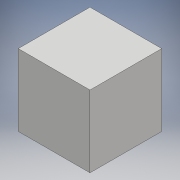
# Autodesk Inventor part: CalibrationCube
Saved by Autodesk Inventor 2017 (Build 210142000, 142)
## iProperties
Created: 2018-12-06
Part Number: CalibrationCube
Material: Generic
Document SubType Name: Modeling
Designer: Eric the Great
Density: 1 g/cm^3
Appearance: Default
Author: Eric the Great
Autodesk Inventor part; units mm, degrees
ref_plane "YZ Plane" through (0, 0, 0) normal (1, 0, 0) x (0, 1, 0)
ref_plane "XZ Plane" through (0, 0, 0) normal (0, 1, 0) x (-1, 0, 0)
ref_plane "XY Plane" through (0, 0, 0) normal (0, 0, 1) x (1, 0, 0)
sketch "Sketch1" plane through (0, 0, 0) normal (0, 1, 0) x (-1, 0, 0)
  line L0 (-28.325, 28.325) -> (28.325, 28.325)
  line L1 (28.325, 28.325) -> (28.325, -28.325)
  line L2 (28.325, -28.325) -> (-28.325, -28.325)
  line L3 (-28.325, -28.325) -> (-28.325, 28.325)
  line L4 (-28.325, 28.325) -> (28.325, -28.325) construction
  line L5 (28.325, 28.325) -> (-28.325, -28.325) construction
  point P0 (0, 0)
  dimension "d1" = 56.65
  constraints: 12 end point, 2 midpoint, 2 parallel, 2 perpendicular, 1 horizontal
  measures "d1" distance of L0.end L1.end
extrude "Extrusion1" add sketch "Sketch1" along normal blind 56.65
sketch "Sketch2" plane through (0, 56.65, 0) normal (0, 1, 0) x (1, 0, 0)
  line L0 (-12.2741, -17.9438) -> (-12.2741, 26.8853) construction
  line L1 (-12.2741, 26.8853) -> (-6.3057, 26.8853) construction
  line L2 (-6.3057, 26.8853) -> (-6.3057, -17.9438) construction
  line L3 (-6.3057, -17.9438) -> (-12.2741, -17.9438) construction
  line L4 (-0.0592, -21.5544) -> (-0.0592, 23.2747) construction
  line L5 (-0.0592, 23.2747) -> (5.9092, 23.2747) construction
  line L6 (5.9092, 23.2747) -> (5.9092, -21.5544) construction
  line L7 (5.9092, -21.5544) -> (-0.0592, -21.5544) construction
  line L8 (-6.8824, -13.4747) -> (-6.8824, -14.3929)
  line L9 (-6.8824, -14.3929) -> (-9.0147, -15.8246)
  line L10 (-9.0147, -15.8246) -> (-9.0147, -16.5513)
  line L11 (-9.0147, -16.5513) -> (-6.8824, -16.5513)
  line L12 (-6.8824, -16.5513) -> (-6.8824, -17.2954)
  line L13 (-6.8824, -17.2954) -> (-11.8824, -17.2954)
  line L14 (-11.8824, -17.2954) -> (-11.8824, -15.5417)
  spline S0 degree 2 poles (-11.8824, -15.5417) (-11.8824, -14.6018) (-11.5038, -13.7837) (-10.9033, -13.7837) knots 0 0 0 1 2 2 2
  line L15 (-10.9033, -13.7837) -> (-10.0417, -13.7837)
  spline S1 degree 2 poles (-10.0417, -13.7837) (-9.5804, -13.7837) (-9.1105, -14.5409) (-9.1105, -15.0805) knots 0 0 0 1 2 2 2
  line L16 (-9.1105, -15.0805) -> (-6.8824, -13.4747)
  line L17 (-10.1331, -14.5322) -> (-10.825, -14.5322)
  spline S2 degree 2 poles (-10.825, -14.5322) (-11.3864, -14.5322) (-11.3864, -15.5026) knots 0 0 0 1 1 1
  line L18 (-11.3864, -15.5026) -> (-11.3864, -16.5513)
  line L19 (-11.3864, -16.5513) -> (-9.5108, -16.5513)
  line L20 (-9.5108, -16.5513) -> (-9.5108, -15.5722)
  spline S3 degree 2 poles (-9.5108, -15.5722) (-9.5108, -15.0413) (-9.7719, -14.5322) (-10.1331, -14.5322) knots 0 0 0 1 2 2 2
  line L21 (-9.3541, -9.332) -> (-8.0617, -9.332)
  spline S4 degree 2 poles (-8.0617, -9.332) (-7.7136, -9.332) (-7.2349, -9.5017) (-6.9738, -9.7628) (-6.8346, -10.2502) (-6.8041, -10.6897) (-6.8041, -11.0509) knots 0 0 0 1 2 3 4 5 5 5
  spline S5 degree 2 poles (-6.8041, -11.0509) (-6.8041, -11.5122) (-6.865, -12.03) (-7.1044, -12.5435) (-7.6309, -12.7698) (-8.0617, -12.7698) knots 0 0 0 1 2 3 4 4 4
  line L22 (-8.0617, -12.7698) -> (-9.3541, -12.7698)
  spline S6 degree 2 poles (-9.3541, -12.7698) (-9.724, -12.7698) (-10.2332, -12.5914) (-10.5117, -12.339) (-10.6553, -11.8429) (-10.6857, -11.4208) (-10.6857, -10.681) (-10.6553, -10.2589) (-10.5117, -9.7628) (-10.2332, -9.5104) (-9.724, -9.332) (-9.3541, -9.332) knots 0 0 0 1 2 3 4 5 6 7 8 9 10 10 10
  line L23 (-7.9616, -10.0413) -> (-9.4716, -10.0413)
  spline S7 degree 2 poles (-9.4716, -10.0413) (-9.9851, -10.0413) (-10.2332, -10.4591) (-10.2332, -11.6427) (-9.9851, -12.0605) (-9.4716, -12.0605) knots 0 0 0 1 2 3 4 4 4
  line L24 (-9.4716, -12.0605) -> (-7.9616, -12.0605)
  spline S8 degree 2 poles (-7.9616, -12.0605) (-7.7136, -12.0605) (-7.422, -11.9517) (-7.2915, -11.6601) (-7.261, -11.3511) (-7.261, -10.7506) (-7.2915, -10.4417) (-7.422, -10.1501) (-7.7136, -10.0413) (-7.9616, -10.0413) knots 0 0 0 1 2 3 4 5 6 7 8 8 8
  line L25 (-9.6327, -4.8585) -> (-8.1009, -4.8585)
  spline S9 degree 2 poles (-8.1009, -4.8585) (-7.7615, -4.8585) (-7.2697, -5.0587) (-6.9999, -5.359) (-6.8433, -5.8551) (-6.8041, -6.2859) (-6.8041, -6.5948) knots 0 0 0 1 2 3 4 5 5 5
  spline S10 degree 2 poles (-6.8041, -6.5948) (-6.8041, -6.9952) (-6.8824, -7.5) (-7.1305, -8.0091) (-7.6744, -8.2571) (-8.1009, -8.2571) knots 0 0 0 1 2 3 4 4 4
  line L26 (-8.1009, -8.2571) -> (-12.2741, -8.2571)
  line L27 (-12.2741, -8.2571) -> (-12.2741, -7.5652)
  line L28 (-12.2741, -7.5652) -> (-11.1557, -7.5652)
  spline S11 degree 2 poles (-11.1557, -7.5652) (-11.0121, -7.5652) (-10.4159, -7.5696) (-10.2723, -7.5696) knots 0 0 0 1 2 2 2
  spline S12 degree 2 poles (-10.2723, -7.5696) (-10.4508, -7.5391) (-10.6857, -6.9647) (-10.6857, -6.399) knots 0 0 0 1 2 2 2
  spline S13 degree 2 poles (-10.6857, -6.399) (-10.6857, -4.8585) (-9.6327, -4.8585) knots 0 0 0 1 1 1
  line L29 (-8.0008, -5.5679) -> (-9.4629, -5.5679)
  spline S14 degree 2 poles (-9.4629, -5.5679) (-9.9416, -5.5679) (-10.194, -6.0161) (-10.194, -6.5861) knots 0 0 0 1 2 2 2
  spline S15 degree 2 poles (-10.194, -6.5861) (-10.194, -7.1344) (-9.9025, -7.5652) (-9.4629, -7.5652) knots 0 0 0 1 2 2 2
  line L30 (-9.4629, -7.5652) -> (-8.0008, -7.5652)
  spline S16 degree 2 poles (-8.0008, -7.5652) (-7.5308, -7.5652) (-7.261, -7.1388) (-7.261, -6.5774) knots 0 0 0 1 2 2 2
  spline S17 degree 2 poles (-7.261, -6.5774) (-7.261, -6.0074) (-7.5308, -5.5679) (-8.0008, -5.5679) knots 0 0 0 1 2 2 2
  line L31 (-9.3541, -0.4982) -> (-8.0617, -0.4982)
  spline S18 degree 2 poles (-8.0617, -0.4982) (-7.7136, -0.4982) (-7.2349, -0.6679) (-6.9738, -0.929) (-6.8346, -1.4164) (-6.8041, -1.8559) (-6.8041, -2.2171) knots 0 0 0 1 2 3 4 5 5 5
  spline S19 degree 2 poles (-6.8041, -2.2171) (-6.8041, -2.6784) (-6.865, -3.1962) (-7.1044, -3.7097) (-7.6309, -3.936) (-8.0617, -3.936) knots 0 0 0 1 2 3 4 4 4
  line L32 (-8.0617, -3.936) -> (-9.3541, -3.936)
  spline S20 degree 2 poles (-9.3541, -3.936) (-9.724, -3.936) (-10.2332, -3.7576) (-10.5117, -3.5052) (-10.6553, -3.0091) (-10.6857, -2.587) (-10.6857, -1.8472) (-10.6553, -1.4251) (-10.5117, -0.929) (-10.2332, -0.6766) (-9.724, -0.4982) (-9.3541, -0.4982) knots 0 0 0 1 2 3 4 5 6 7 8 9 10 10 10
  line L33 (-7.9616, -1.2075) -> (-9.4716, -1.2075)
  spline S21 degree 2 poles (-9.4716, -1.2075) (-9.9851, -1.2075) (-10.2332, -1.6253) (-10.2332, -2.8089) (-9.9851, -3.2267) (-9.4716, -3.2267) knots 0 0 0 1 2 3 4 4 4
  line L34 (-9.4716, -3.2267) -> (-7.9616, -3.2267)
  spline S22 degree 2 poles (-7.9616, -3.2267) (-7.7136, -3.2267) (-7.422, -3.1179) (-7.2915, -2.8263) (-7.261, -2.5174) (-7.261, -1.9169) (-7.2915, -1.6079) (-7.422, -1.3163) (-7.7136, -1.2075) (-7.9616, -1.2075) knots 0 0 0 1 2 3 4 5 6 7 8 8 8
  spline S23 degree 2 poles (-6.9129, 3.2746) (-6.8041, 2.7655) (-6.8041, 2.0779) knots 0 0 0 1 1 1
  spline S24 degree 2 poles (-6.8041, 2.0779) (-6.8041, 1.7385) (-6.8302, 1.3643) (-6.9608, 0.8769) (-7.2045, 0.6245) (-7.6744, 0.4374) (-8.0226, 0.4374) knots 0 0 0 1 2 3 4 5 5 5
  line L35 (-8.0226, 0.4374) -> (-9.3933, 0.4374)
  spline S25 degree 2 poles (-9.3933, 0.4374) (-9.7023, 0.4374) (-10.1461, 0.5549) (-10.4246, 0.7986) (-10.5944, 1.064) (-10.664, 1.5166) (-10.6857, 1.8647) (-10.6857, 2.1563) knots 0 0 0 1 2 3 4 5 6 6 6
  spline S26 degree 2 poles (-10.6857, 2.1563) (-10.6857, 2.6872) (-10.5726, 3.218) knots 0 0 0 1 1 1
  line L36 (-10.5726, 3.218) -> (-10.0635, 3.218)
  spline S27 degree 2 poles (-10.0635, 3.218) (-10.2158, 2.6175) (-10.2158, 2.0692) knots 0 0 0 1 1 1
  spline S28 degree 2 poles (-10.2158, 2.0692) (-10.2158, 1.4948) (-9.9416, 1.1467) (-9.4934, 1.1467) knots 0 0 0 1 2 2 2
  line L37 (-9.4934, 1.1467) -> (-7.9703, 1.1467)
  spline S29 degree 2 poles (-7.9703, 1.1467) (-7.5613, 1.1467) (-7.2915, 1.5383) (-7.2915, 2.1476) knots 0 0 0 1 2 2 2
  spline S30 degree 2 poles (-7.2915, 2.1476) (-7.2915, 2.6959) (-7.4351, 3.2746) knots 0 0 0 1 1 1
  line L38 (-7.4351, 3.2746) -> (-6.9129, 3.2746)
  line L39 (-6.8824, 7.3608) -> (-6.8824, 6.6689)
  line L40 (-6.8824, 6.6689) -> (-7.335, 6.6689)
  spline S31 degree 2 poles (-7.335, 6.6689) (-6.8041, 6.5601) (-6.8041, 5.4417) knots 0 0 0 1 1 1
  spline S32 degree 2 poles (-6.8041, 5.4417) (-6.8041, 4.7063) (-7.335, 4.1493) (-7.8746, 4.1493) knots 0 0 0 1 2 2 2
  line L41 (-7.8746, 4.1493) -> (-10.6118, 4.1493)
  line L42 (-10.6118, 4.1493) -> (-10.6118, 4.8412)
  line L43 (-10.6118, 4.8412) -> (-7.9138, 4.8412)
  spline S33 degree 2 poles (-7.9138, 4.8412) (-7.7745, 4.8412) (-7.5917, 4.8891) (-7.4003, 5.037) (-7.3002, 5.3808) (-7.3002, 5.6419) knots 0 0 0 1 2 3 4 4 4
  spline S34 degree 2 poles (-7.3002, 5.6419) (-7.3002, 6.2207) (-7.5134, 6.6689) (-7.8006, 6.6689) knots 0 0 0 1 2 2 2
  line L44 (-7.8006, 6.6689) -> (-10.6118, 6.6689)
  line L45 (-10.6118, 6.6689) -> (-10.6118, 7.3608)
  line L46 (-10.6118, 7.3608) -> (-6.8824, 7.3608)
  line L47 (-9.6327, 11.9604) -> (-8.1009, 11.9604)
  spline S35 degree 2 poles (-8.1009, 11.9604) (-7.7615, 11.9604) (-7.2697, 11.7603) (-6.9999, 11.46) (-6.8433, 10.9639) (-6.8041, 10.5331) (-6.8041, 10.2241) knots 0 0 0 1 2 3 4 5 5 5
  spline S36 degree 2 poles (-6.8041, 10.2241) (-6.8041, 9.8238) (-6.8824, 9.319) (-7.1305, 8.8099) (-7.6744, 8.5618) (-8.1009, 8.5618) knots 0 0 0 1 2 3 4 4 4
  line L48 (-8.1009, 8.5618) -> (-12.2741, 8.5618)
  line L49 (-12.2741, 8.5618) -> (-12.2741, 9.2537)
  line L50 (-12.2741, 9.2537) -> (-11.1557, 9.2537)
  spline S37 degree 2 poles (-11.1557, 9.2537) (-11.0121, 9.2537) (-10.4159, 9.2494) (-10.2723, 9.2494) knots 0 0 0 1 2 2 2
  spline S38 degree 2 poles (-10.2723, 9.2494) (-10.4508, 9.2798) (-10.6857, 9.8543) (-10.6857, 10.42) knots 0 0 0 1 2 2 2
  spline S39 degree 2 poles (-10.6857, 10.42) (-10.6857, 11.9604) (-9.6327, 11.9604) knots 0 0 0 1 1 1
  line L51 (-8.0008, 11.2511) -> (-9.4629, 11.2511)
  spline S40 degree 2 poles (-9.4629, 11.2511) (-9.9416, 11.2511) (-10.194, 10.8029) (-10.194, 10.2328) knots 0 0 0 1 2 2 2
  spline S41 degree 2 poles (-10.194, 10.2328) (-10.194, 9.6845) (-9.9025, 9.2537) (-9.4629, 9.2537) knots 0 0 0 1 2 2 2
  line L52 (-9.4629, 9.2537) -> (-8.0008, 9.2537)
  spline S42 degree 2 poles (-8.0008, 9.2537) (-7.5308, 9.2537) (-7.261, 9.6802) (-7.261, 10.2415) knots 0 0 0 1 2 2 2
  spline S43 degree 2 poles (-7.261, 10.2415) (-7.261, 10.8116) (-7.5308, 11.2511) (-8.0008, 11.2511) knots 0 0 0 1 2 2 2
  line L53 (-8.5926, 16.0901) -> (-8.5926, 13.5836)
  line L54 (-8.5926, 13.5836) -> (-8.0313, 13.5836)
  spline S44 degree 2 poles (-8.0313, 13.5836) (-7.6353, 13.5836) (-7.3045, 14.1406) (-7.3045, 14.6845) knots 0 0 0 1 2 2 2
  spline S45 degree 2 poles (-7.3045, 14.6845) (-7.3045, 15.2198) (-7.4917, 15.9422) knots 0 0 0 1 1 1
  line L55 (-7.4917, 15.9422) -> (-6.9608, 15.9422)
  spline S46 degree 2 poles (-6.9608, 15.9422) (-6.8041, 15.2502) (-6.8041, 14.5932) knots 0 0 0 1 1 1
  spline S47 degree 2 poles (-6.8041, 14.5932) (-6.8041, 12.883) (-7.9442, 12.883) knots 0 0 0 1 1 1
  line L56 (-7.9442, 12.883) -> (-9.4151, 12.883)
  spline S48 degree 2 poles (-9.4151, 12.883) (-10.1026, 12.883) (-10.6857, 13.6706) (-10.6857, 14.5322) knots 0 0 0 1 2 2 2
  spline S49 degree 2 poles (-10.6857, 14.5322) (-10.6857, 15.3416) (-10.1244, 16.0901) (-9.4151, 16.0901) knots 0 0 0 1 2 2 2
  line L57 (-9.4151, 16.0901) -> (-8.5926, 16.0901)
  line L58 (-9.0452, 15.3939) -> (-9.6327, 15.3939)
  spline S50 degree 2 poles (-9.6327, 15.3939) (-9.9721, 15.3939) (-10.2245, 14.9804) (-10.2245, 14.4931) knots 0 0 0 1 2 2 2
  spline S51 degree 2 poles (-10.2245, 14.4931) (-10.2245, 14.0318) (-9.9808, 13.5836) (-9.6327, 13.5836) knots 0 0 0 1 2 2 2
  line L59 (-9.6327, 13.5836) -> (-9.0452, 13.5836)
  line L60 (-9.0452, 13.5836) -> (-9.0452, 15.3939)
  line L61 (1.5257, 0.3275) -> (2.4447, 0.3275)
  spline S52 degree 2 poles (2.4447, 0.3275) (2.6484, 0.3275) (2.9434, 0.2074) (3.1053, 0.0273) (3.1993, -0.2704) (3.2228, -0.5289) (3.2228, -0.7142) knots 0 0 0 1 2 3 4 5 5 5
  spline S53 degree 2 poles (3.2228, -0.7142) (3.2228, -0.9545) (3.1758, -1.2573) (3.027, -1.5628) (2.7006, -1.7116) (2.4447, -1.7116) knots 0 0 0 1 2 3 4 4 4
  line L62 (2.4447, -1.7116) -> (-0.0592, -1.7116)
  line L63 (-0.0592, -1.7116) -> (-0.0592, -1.2965)
  line L64 (-0.0592, -1.2965) -> (0.6118, -1.2965)
  spline S54 degree 2 poles (0.6118, -1.2965) (0.698, -1.2965) (1.0557, -1.2991) (1.1419, -1.2991) knots 0 0 0 1 2 2 2
  spline S55 degree 2 poles (1.1419, -1.2991) (1.0348, -1.2808) (0.8938, -0.9362) (0.8938, -0.5968) knots 0 0 0 1 2 2 2
  spline S56 degree 2 poles (0.8938, -0.5968) (0.8938, 0.3275) (1.5257, 0.3275) knots 0 0 0 1 1 1
  line L65 (2.5048, -0.0981) -> (1.6275, -0.0981)
  spline S57 degree 2 poles (1.6275, -0.0981) (1.3403, -0.0981) (1.1889, -0.367) (1.1889, -0.709) knots 0 0 0 1 2 2 2
  spline S58 degree 2 poles (1.1889, -0.709) (1.1889, -1.038) (1.3638, -1.2965) (1.6275, -1.2965) knots 0 0 0 1 2 2 2
  line L66 (1.6275, -1.2965) -> (2.5048, -1.2965)
  spline S59 degree 2 poles (2.5048, -1.2965) (2.7868, -1.2965) (2.9486, -1.0406) (2.9486, -0.7038) knots 0 0 0 1 2 2 2
  spline S60 degree 2 poles (2.9486, -0.7038) (2.9486, -0.3618) (2.7868, -0.0981) (2.5048, -0.0981) knots 0 0 0 1 2 2 2
  line L67 (0.9382, 2.7035) -> (4.1366, 1.5782)
  line L68 (4.1366, 1.5782) -> (4.1366, 1.1448)
  line L69 (4.1366, 1.1448) -> (3.2071, 1.4972)
  line L70 (3.2071, 1.4972) -> (0.9382, 0.633)
  line L71 (0.9382, 0.633) -> (0.9382, 1.0847)
  line L72 (0.9382, 1.0847) -> (2.7633, 1.7087)
  line L73 (2.7633, 1.7087) -> (2.7633, 1.7192)
  line L74 (2.7633, 1.7192) -> (0.9382, 2.2831)
  line L75 (0.9382, 2.2831) -> (0.9382, 2.7035)
  line L76 (7.9851, -8.6868) -> (7.9851, -9.2377)
  line L77 (7.9851, -9.2377) -> (6.7058, -10.0968)
  line L78 (6.7058, -10.0968) -> (6.7058, -10.5328)
  line L79 (6.7058, -10.5328) -> (7.9851, -10.5328)
  line L80 (7.9851, -10.5328) -> (7.9851, -10.9793)
  line L81 (7.9851, -10.9793) -> (4.9851, -10.9793)
  line L82 (4.9851, -10.9793) -> (4.9851, -9.927)
  spline S61 degree 2 poles (4.9851, -9.927) (4.9851, -9.3631) (5.2123, -8.8722) (5.5726, -8.8722) knots 0 0 0 1 2 2 2
  line L83 (5.5726, -8.8722) -> (6.0896, -8.8722)
  spline S62 degree 2 poles (6.0896, -8.8722) (6.3663, -8.8722) (6.6483, -9.3265) (6.6483, -9.6503) knots 0 0 0 1 2 2 2
  line L84 (6.6483, -9.6503) -> (7.9851, -8.6868)
  line L85 (6.0348, -9.3213) -> (5.6196, -9.3213)
  spline S63 degree 2 poles (5.6196, -9.3213) (5.2828, -9.3213) (5.2828, -9.9035) knots 0 0 0 1 1 1
  line L86 (5.2828, -9.9035) -> (5.2828, -10.5328)
  line L87 (5.2828, -10.5328) -> (6.4081, -10.5328)
  line L88 (6.4081, -10.5328) -> (6.4081, -9.9453)
  spline S64 degree 2 poles (6.4081, -9.9453) (6.4081, -9.6268) (6.2515, -9.3213) (6.0348, -9.3213) knots 0 0 0 1 2 2 2
  line L89 (6.5021, -6.2012) -> (7.2776, -6.2012)
  spline S65 degree 2 poles (7.2776, -6.2012) (7.4864, -6.2012) (7.7737, -6.303) (7.9303, -6.4597) (8.0139, -6.7521) (8.0321, -7.0158) (8.0321, -7.2325) knots 0 0 0 1 2 3 4 5 5 5
  spline S66 degree 2 poles (8.0321, -7.2325) (8.0321, -7.5093) (7.9956, -7.82) (7.852, -8.1281) (7.5361, -8.2639) (7.2776, -8.2639) knots 0 0 0 1 2 3 4 4 4
  line L90 (7.2776, -8.2639) -> (6.5021, -8.2639)
  spline S67 degree 2 poles (6.5021, -8.2639) (6.2802, -8.2639) (5.9747, -8.1568) (5.8076, -8.0054) (5.7214, -7.7077) (5.7032, -7.4545) (5.7032, -7.0106) (5.7214, -6.7573) (5.8076, -6.4597) (5.9747, -6.3082) (6.2802, -6.2012) (6.5021, -6.2012) knots 0 0 0 1 2 3 4 5 6 7 8 9 10 10 10
  line L91 (7.3376, -6.6268) -> (6.4316, -6.6268)
  spline S68 degree 2 poles (6.4316, -6.6268) (6.1235, -6.6268) (5.9747, -6.8774) (5.9747, -7.5876) (6.1235, -7.8383) (6.4316, -7.8383) knots 0 0 0 1 2 3 4 4 4
  line L92 (6.4316, -7.8383) -> (7.3376, -7.8383)
  spline S69 degree 2 poles (7.3376, -7.8383) (7.4864, -7.8383) (7.6614, -7.773) (7.7397, -7.5981) (7.758, -7.4127) (7.758, -7.0524) (7.7397, -6.867) (7.6614, -6.6921) (7.4864, -6.6268) (7.3376, -6.6268) knots 0 0 0 1 2 3 4 5 6 7 8 8 8
  line L93 (7.9851, -3.6294) -> (7.9851, -4.0445)
  line L94 (7.9851, -4.0445) -> (6.3663, -4.0445)
  spline S70 degree 2 poles (6.3663, -4.0445) (6.2854, -4.0445) (6.1731, -4.0733) (6.0583, -4.1594) (5.9982, -4.3683) (5.9982, -4.525) knots 0 0 0 1 2 3 4 4 4
  spline S71 degree 2 poles (5.9982, -4.525) (5.9982, -4.8905) (6.1549, -5.1411) (6.3663, -5.1411) knots 0 0 0 1 2 2 2
  line L95 (6.3663, -5.1411) -> (7.9851, -5.1411)
  line L96 (7.9851, -5.1411) -> (7.9851, -5.5563)
  line L97 (7.9851, -5.5563) -> (5.7475, -5.5563)
  line L98 (5.7475, -5.5563) -> (5.7475, -5.1411)
  line L99 (5.7475, -5.1411) -> (6.0217, -5.1411)
  spline S72 degree 2 poles (6.0217, -5.1411) (5.7032, -5.0759) (5.7032, -4.4048) knots 0 0 0 1 1 1
  spline S73 degree 2 poles (5.7032, -4.4048) (5.7032, -3.961) (6.0217, -3.6294) (6.3455, -3.6294) knots 0 0 0 1 2 2 2
  line L100 (6.3455, -3.6294) -> (7.9851, -3.6294)
  line L101 (6.335, -0.8696) -> (7.2541, -0.8696)
  spline S74 degree 2 poles (7.2541, -0.8696) (7.4577, -0.8696) (7.7528, -0.9897) (7.9146, -1.1699) (8.0086, -1.4675) (8.0321, -1.726) (8.0321, -1.9114) knots 0 0 0 1 2 3 4 5 5 5
  spline S75 degree 2 poles (8.0321, -1.9114) (8.0321, -2.1516) (7.9851, -2.4545) (7.8363, -2.7599) (7.5099, -2.9088) (7.2541, -2.9088) knots 0 0 0 1 2 3 4 4 4
  line L102 (7.2541, -2.9088) -> (4.7502, -2.9088)
  line L103 (4.7502, -2.9088) -> (4.7502, -2.4936)
  line L104 (4.7502, -2.4936) -> (5.4212, -2.4936)
  spline S76 degree 2 poles (5.4212, -2.4936) (5.5073, -2.4936) (5.865, -2.4962) (5.9512, -2.4962) knots 0 0 0 1 2 2 2
  spline S77 degree 2 poles (5.9512, -2.4962) (5.8442, -2.478) (5.7032, -2.1333) (5.7032, -1.7939) knots 0 0 0 1 2 2 2
  spline S78 degree 2 poles (5.7032, -1.7939) (5.7032, -0.8696) (6.335, -0.8696) knots 0 0 0 1 1 1
  line L105 (7.3141, -1.2952) -> (6.4368, -1.2952)
  spline S79 degree 2 poles (6.4368, -1.2952) (6.1496, -1.2952) (5.9982, -1.5641) (5.9982, -1.9062) knots 0 0 0 1 2 2 2
  spline S80 degree 2 poles (5.9982, -1.9062) (5.9982, -2.2351) (6.1731, -2.4936) (6.4368, -2.4936) knots 0 0 0 1 2 2 2
  line L106 (6.4368, -2.4936) -> (7.3141, -2.4936)
  spline S81 degree 2 poles (7.3141, -2.4936) (7.5961, -2.4936) (7.758, -2.2377) (7.758, -1.9009) knots 0 0 0 1 2 2 2
  spline S82 degree 2 poles (7.758, -1.9009) (7.758, -1.5589) (7.5961, -1.2952) (7.3141, -1.2952) knots 0 0 0 1 2 2 2
  line L107 (6.959, 1.6082) -> (6.959, 0.1043)
  line L108 (6.959, 0.1043) -> (7.2958, 0.1043)
  spline S83 degree 2 poles (7.2958, 0.1043) (7.5334, 0.1043) (7.7319, 0.4385) (7.7319, 0.7649) knots 0 0 0 1 2 2 2
  spline S84 degree 2 poles (7.7319, 0.7649) (7.7319, 1.086) (7.6196, 1.5194) knots 0 0 0 1 1 1
  line L109 (7.6196, 1.5194) -> (7.9381, 1.5194)
  spline S85 degree 2 poles (7.9381, 1.5194) (8.0321, 1.1043) (8.0321, 0.71) knots 0 0 0 1 1 1
  spline S86 degree 2 poles (8.0321, 0.71) (8.0321, -0.3161) (7.3481, -0.3161) knots 0 0 0 1 1 1
  line L110 (7.3481, -0.3161) -> (6.4656, -0.3161)
  spline S87 degree 2 poles (6.4656, -0.3161) (6.053, -0.3161) (5.7032, 0.1565) (5.7032, 0.6735) knots 0 0 0 1 2 2 2
  spline S88 degree 2 poles (5.7032, 0.6735) (5.7032, 1.1591) (6.04, 1.6082) (6.4656, 1.6082) knots 0 0 0 1 2 2 2
  line L111 (6.4656, 1.6082) -> (6.959, 1.6082)
  line L112 (6.6875, 1.1905) -> (6.335, 1.1905)
  spline S89 degree 2 poles (6.335, 1.1905) (6.1314, 1.1905) (5.9799, 0.9424) (5.9799, 0.65) knots 0 0 0 1 2 2 2
  spline S90 degree 2 poles (5.9799, 0.65) (5.9799, 0.3732) (6.1261, 0.1043) (6.335, 0.1043) knots 0 0 0 1 2 2 2
  line L113 (6.335, 0.1043) -> (6.6875, 0.1043)
  line L114 (6.6875, 0.1043) -> (6.6875, 1.1905)
  line L115 (6.0583, 3.4463) -> (6.0583, 3.2166)
  spline S91 degree 2 poles (6.0583, 3.2166) (6.0583, 2.9294) (6.2071, 2.6552) (6.4081, 2.6552) knots 0 0 0 1 2 2 2
  line L116 (6.4081, 2.6552) -> (7.9851, 2.6552)
  line L117 (7.9851, 2.6552) -> (7.9851, 2.2401)
  line L118 (7.9851, 2.2401) -> (5.7475, 2.2401)
  line L119 (5.7475, 2.2401) -> (5.7475, 2.6343)
  line L120 (5.7475, 2.6343) -> (6.1131, 2.6343)
  spline S92 degree 2 poles (6.1131, 2.6343) (5.9512, 2.6343) (5.7032, 3.0364) (5.7032, 3.2427) knots 0 0 0 1 2 2 2
  line L121 (5.7032, 3.2427) -> (5.7032, 3.4463)
  line L122 (5.7032, 3.4463) -> (6.0583, 3.4463)
  line L123 (5.7475, 5.7701) -> (8.1966, 5.7701)
  spline S93 degree 2 poles (8.1966, 5.7701) (8.6744, 5.7701) (9.0008, 5.2401) (9.0008, 4.7074) knots 0 0 0 1 2 2 2
  spline S94 degree 2 poles (9.0008, 4.7074) (9.0008, 4.2322) (8.9512, 3.9346) knots 0 0 0 1 1 1
  line L124 (8.9512, 3.9346) -> (8.6562, 3.9346)
  spline S95 degree 2 poles (8.6562, 3.9346) (8.7188, 4.4672) (8.7188, 4.744) knots 0 0 0 1 1 1
  spline S96 degree 2 poles (8.7188, 4.744) (8.7188, 5.0625) (8.5178, 5.3549) (8.2802, 5.3549) knots 0 0 0 1 2 2 2
  line L125 (8.2802, 5.3549) -> (7.7449, 5.3549)
  spline S97 degree 2 poles (7.7449, 5.3549) (7.9016, 5.3445) (8.0321, 4.9346) (8.0321, 4.6709) knots 0 0 0 1 2 2 2
  spline S98 degree 2 poles (8.0321, 4.6709) (8.0321, 4.1539) (7.7267, 3.7779) (7.3533, 3.7779) knots 0 0 0 1 2 2 2
  line L126 (7.3533, 3.7779) -> (6.4421, 3.7779)
  spline S99 degree 2 poles (6.4421, 3.7779) (6.0452, 3.7779) (5.7032, 4.2087) (5.7032, 4.697) knots 0 0 0 1 2 2 2
  spline S100 degree 2 poles (5.7032, 4.697) (5.7032, 5.2792) (5.9669, 5.3811) knots 0 0 0 1 1 1
  line L127 (5.9669, 5.3811) -> (5.7475, 5.3811)
  line L128 (5.7475, 5.3811) -> (5.7475, 5.7701)
  line L129 (7.3794, 5.3549) -> (6.3663, 5.3549)
  spline S101 degree 2 poles (6.3663, 5.3549) (6.1496, 5.3549) (5.9878, 5.12) (5.9878, 4.7492) knots 0 0 0 1 2 2 2
  spline S102 degree 2 poles (5.9878, 4.7492) (5.9878, 4.4019) (6.147, 4.1905) (6.3663, 4.1905) knots 0 0 0 1 2 2 2
  line L130 (6.3663, 4.1905) -> (7.3794, 4.1905)
  spline S103 degree 2 poles (7.3794, 4.1905) (7.6118, 4.1905) (7.7528, 4.415) (7.7528, 4.757) knots 0 0 0 1 2 2 2
  spline S104 degree 2 poles (7.7528, 4.757) (7.7528, 5.073) (7.6013, 5.3549) (7.3794, 5.3549) knots 0 0 0 1 2 2 2
  line L131 (5.7475, 8.2296) -> (8.946, 7.1043)
  line L132 (8.946, 7.1043) -> (8.946, 6.6709)
  line L133 (8.946, 6.6709) -> (8.0165, 7.0234)
  line L134 (8.0165, 7.0234) -> (5.7475, 6.1591)
  line L135 (5.7475, 6.1591) -> (5.7475, 6.6108)
  line L136 (5.7475, 6.6108) -> (7.5726, 7.2348)
  line L137 (7.5726, 7.2348) -> (7.5726, 7.2453)
  line L138 (7.5726, 7.2453) -> (5.7475, 7.8093)
  line L139 (5.7475, 7.8093) -> (5.7475, 8.2296)
  line L140 (5.5778, 11.744) -> (6.2019, 11.744)
  spline S105 degree 2 poles (6.2019, 11.744) (6.5857, 11.744) (6.9042, 11.1487) (6.9042, 10.603) knots 0 0 0 1 2 2 2
  line L141 (6.9042, 10.603) -> (6.9042, 10.1539)
  line L142 (6.9042, 10.1539) -> (7.9851, 10.1539)
  line L143 (7.9851, 10.1539) -> (7.9851, 9.7074)
  line L144 (7.9851, 9.7074) -> (4.9851, 9.7074)
  line L145 (4.9851, 9.7074) -> (4.9851, 10.6865)
  spline S106 degree 2 poles (4.9851, 10.6865) (4.9851, 10.8719) (5.0034, 11.1382) (5.0739, 11.4385) (5.1992, 11.6187) (5.4212, 11.744) (5.5778, 11.744) knots 0 0 0 1 2 3 4 5 5 5
  line L146 (6.1784, 11.3053) -> (5.6327, 11.3053)
  spline S107 degree 2 poles (5.6327, 11.3053) (5.5073, 11.3053) (5.3455, 11.1774) (5.2828, 10.9372) (5.2671, 10.7753) (5.2671, 10.6552) knots 0 0 0 1 2 3 4 4 4
  line L147 (5.2671, 10.6552) -> (5.2671, 10.1513)
  line L148 (5.2671, 10.1513) -> (6.6222, 10.1513)
  line L149 (6.6222, 10.1513) -> (6.6222, 10.663)
  spline S108 degree 2 poles (6.6222, 10.663) (6.6222, 10.932) (6.4238, 11.3053) (6.1784, 11.3053) knots 0 0 0 1 2 2 2
  line L150 (7.9851, 12.7283) -> (7.9851, 12.3132)
  line L151 (7.9851, 12.3132) -> (5.7475, 12.3132)
  line L152 (5.7475, 12.3132) -> (5.7475, 12.7283)
  line L153 (5.7475, 12.7283) -> (7.9851, 12.7283)
  line L154 (5.3742, 12.7283) -> (5.3742, 12.3132)
  line L155 (5.3742, 12.3132) -> (4.9408, 12.3132)
  line L156 (4.9408, 12.3132) -> (4.9408, 12.7283)
  line L157 (4.9408, 12.7283) -> (5.3742, 12.7283)
  point P0 (0, 0)
  constraints: 4 other
extrude "Extrusion2" cut sketch "Sketch2" against normal blind 2
body "Solid1"
